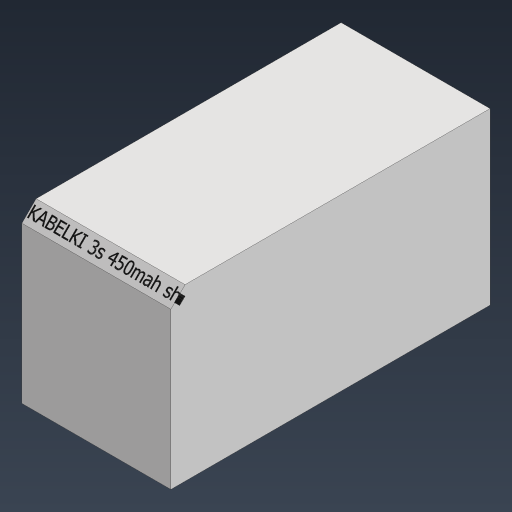
# Autodesk Inventor part: 2s450mah
Saved by Autodesk Inventor 2023 (Build 270158000, 158)
## iProperties
Created: 2026-03-09
Part Number: 2s450mah
Material: Generic
Document SubType Name: Modeling
Designer: szymo
Density: 1 g/cm^3
Appearance: Default
Author: szymo
Autodesk Inventor part; units mm, degrees
ref_plane "YZ Plane" through (0, 0, 0) normal (1, 0, 0) x (0, 1, 0)
ref_plane "XZ Plane" through (0, 0, 0) normal (0, 1, 0) x (-1, 0, 0)
ref_plane "XY Plane" through (0, 0, 0) normal (0, 0, 1) x (1, 0, 0)
sketch "Sketch1" plane through (0, 0, 0) normal (0, 1, 0) x (-1, 0, 0)
  line L0 (0, 0) -> (-21, 0)
  line L1 (-21, 0) -> (-21, -45)
  line L2 (-21, -45) -> (0, -45)
  line L3 (0, -45) -> (0, 0)
  dimension "d0" = 21
  dimension "d1" = 45
  constraints: 8 end point, 2 parallel, 1 horizontal, 1 perpendicular
  measures "d0" distance of L2.end L1.end
  measures "d1" distance of L0.end L1.end
extrude "Extrusion1" add sketch "Sketch1" along normal blind 24
chamfer "Chamfer1" distance 2 angle 45 1 edges at (10.5, 24, 0)
sketch "Sketch2" plane through (0, 24, -2) normal (0, 0.7071068, 0.7071068) x (1, 0, 0)
  line L0 (0.0469, -0.5129) -> (26.4473, -0.5129) construction
  line L1 (26.4473, -0.5129) -> (26.4473, -3.2591) construction
  line L2 (26.4473, -3.2591) -> (0.0469, -3.2591) construction
  line L3 (0.0469, -3.2591) -> (0.0469, -0.5129) construction
  line L4 (1.2929, -2.0798) -> (1.0339, -2.0798)
  line L5 (1.0339, -2.0798) -> (0.4857, -1.382)
  line L6 (0.4857, -1.382) -> (0.3982, -1.4805)
  line L7 (0.3982, -1.4805) -> (0.3982, -2.0798)
  line L8 (0.3982, -2.0798) -> (0.1989, -2.0798)
  line L9 (0.1989, -2.0798) -> (0.1989, -0.5798)
  line L10 (0.1989, -0.5798) -> (0.3982, -0.5798)
  line L11 (0.3982, -0.5798) -> (0.3982, -1.269)
  line L12 (0.3982, -1.269) -> (1.0133, -0.5798)
  line L13 (1.0133, -0.5798) -> (1.2564, -0.5798)
  line L14 (1.2564, -0.5798) -> (0.6352, -1.2495)
  line L15 (0.6352, -1.2495) -> (1.2929, -2.0798)
  line L16 (1.2503, -2.0798) -> (1.756, -0.5798)
  line L17 (1.756, -0.5798) -> (2.0015, -0.5798)
  line L18 (2.0015, -0.5798) -> (2.5072, -2.0798)
  line L19 (2.5072, -2.0798) -> (2.2969, -2.0798)
  line L20 (2.2969, -2.0798) -> (2.1608, -1.6604)
  line L21 (2.1608, -1.6604) -> (1.5882, -1.6604)
  line L22 (1.5882, -1.6604) -> (1.4521, -2.0798)
  line L23 (1.4521, -2.0798) -> (1.2503, -2.0798)
  line L24 (2.1061, -1.4902) -> (1.8739, -0.784)
  line L25 (1.8739, -0.784) -> (1.6429, -1.4902)
  line L26 (1.6429, -1.4902) -> (2.1061, -1.4902)
  spline S0 degree 2 poles (3.6668, -1.6191) (3.6668, -1.7309) (3.5818, -1.9023) (3.5113, -1.9582) knots 0 0 0 1 2 2 2
  spline S1 degree 2 poles (3.5113, -1.9582) (3.4262, -2.0238) (3.2329, -2.0798) (3.0797, -2.0798) knots 0 0 0 1 2 2 2
  line L27 (3.0797, -2.0798) -> (2.6494, -2.0798)
  line L28 (2.6494, -2.0798) -> (2.6494, -0.5798)
  line L29 (2.6494, -0.5798) -> (3.0469, -0.5798)
  spline S2 degree 2 poles (3.0469, -0.5798) (3.2074, -0.5798) (3.3678, -0.6004) (3.4407, -0.6405) knots 0 0 0 1 2 2 2
  spline S3 degree 2 poles (3.4407, -0.6405) (3.5222, -0.6831) (3.5963, -0.8229) (3.5963, -0.9177) knots 0 0 0 1 2 2 2
  spline S4 degree 2 poles (3.5963, -0.9177) (3.5963, -1.0234) (3.4845, -1.1912) (3.386, -1.2386) knots 0 0 0 1 2 2 2
  line L30 (3.386, -1.2386) -> (3.386, -1.2459)
  spline S5 degree 2 poles (3.386, -1.2459) (3.5198, -1.2824) (3.6668, -1.4756) (3.6668, -1.6191) knots 0 0 0 1 2 2 2
  spline S6 degree 2 poles (3.459, -1.6276) (3.459, -1.5425) (3.4104, -1.4331) (3.3374, -1.3942) knots 0 0 0 1 2 2 2
  spline S7 degree 2 poles (3.3374, -1.3942) (3.29, -1.3699) (3.1782, -1.3553) (3.0749, -1.3553) knots 0 0 0 1 2 2 2
  line L31 (3.0749, -1.3553) -> (2.8488, -1.3553)
  line L32 (2.8488, -1.3553) -> (2.8488, -1.9096)
  line L33 (2.8488, -1.9096) -> (3.0104, -1.9096)
  spline S8 degree 2 poles (3.0104, -1.9096) (3.1417, -1.9096) (3.2924, -1.8853) (3.3508, -1.8464) knots 0 0 0 1 2 2 2
  spline S9 degree 2 poles (3.3508, -1.8464) (3.4067, -1.8063) (3.459, -1.7066) (3.459, -1.6276) knots 0 0 0 1 2 2 2
  spline S10 degree 2 poles (3.3885, -0.9456) (3.3885, -0.8922) (3.352, -0.8119) (3.3119, -0.7888) knots 0 0 0 1 2 2 2
  spline S11 degree 2 poles (3.3119, -0.7888) (3.2633, -0.7621) (3.1454, -0.7499) (3.0396, -0.7499) knots 0 0 0 1 2 2 2
  line L34 (3.0396, -0.7499) -> (2.8488, -0.7499)
  line L35 (2.8488, -0.7499) -> (2.8488, -1.1888)
  line L36 (2.8488, -1.1888) -> (3.0749, -1.1888)
  spline S12 degree 2 poles (3.0749, -1.1888) (3.1685, -1.1888) (3.2572, -1.1693) (3.3046, -1.1389) knots 0 0 0 1 2 2 2
  spline S13 degree 2 poles (3.3046, -1.1389) (3.3508, -1.1097) (3.3885, -1.0161) (3.3885, -0.9456) knots 0 0 0 1 2 2 2
  line L37 (3.865, -2.0798) -> (3.865, -0.5798)
  line L38 (3.865, -0.5798) -> (4.8034, -0.5798)
  line L39 (4.8034, -0.5798) -> (4.8034, -0.7572)
  line L40 (4.8034, -0.7572) -> (4.0643, -0.7572)
  line L41 (4.0643, -0.7572) -> (4.0643, -1.1681)
  line L42 (4.0643, -1.1681) -> (4.7536, -1.1681)
  line L43 (4.7536, -1.1681) -> (4.7536, -1.3456)
  line L44 (4.7536, -1.3456) -> (4.0643, -1.3456)
  line L45 (4.0643, -1.3456) -> (4.0643, -1.9023)
  line L46 (4.0643, -1.9023) -> (4.8034, -1.9023)
  line L47 (4.8034, -1.9023) -> (4.8034, -2.0798)
  line L48 (4.8034, -2.0798) -> (3.865, -2.0798)
  line L49 (5.8913, -2.0798) -> (5.0222, -2.0798)
  line L50 (5.0222, -2.0798) -> (5.0222, -0.5798)
  line L51 (5.0222, -0.5798) -> (5.2215, -0.5798)
  line L52 (5.2215, -0.5798) -> (5.2215, -1.9023)
  line L53 (5.2215, -1.9023) -> (5.8913, -1.9023)
  line L54 (5.8913, -1.9023) -> (5.8913, -2.0798)
  line L55 (7.1421, -2.0798) -> (6.8832, -2.0798)
  line L56 (6.8832, -2.0798) -> (6.335, -1.382)
  line L57 (6.335, -1.382) -> (6.2475, -1.4805)
  line L58 (6.2475, -1.4805) -> (6.2475, -2.0798)
  line L59 (6.2475, -2.0798) -> (6.0481, -2.0798)
  line L60 (6.0481, -2.0798) -> (6.0481, -0.5798)
  line L61 (6.0481, -0.5798) -> (6.2475, -0.5798)
  line L62 (6.2475, -0.5798) -> (6.2475, -1.269)
  line L63 (6.2475, -1.269) -> (6.8625, -0.5798)
  line L64 (6.8625, -0.5798) -> (7.1057, -0.5798)
  line L65 (7.1057, -0.5798) -> (6.4845, -1.2495)
  line L66 (6.4845, -1.2495) -> (7.1421, -2.0798)
  line L67 (7.7839, -2.0798) -> (7.2029, -2.0798)
  line L68 (7.2029, -2.0798) -> (7.2029, -1.9266)
  line L69 (7.2029, -1.9266) -> (7.3937, -1.9266)
  line L70 (7.3937, -1.9266) -> (7.3937, -0.7329)
  line L71 (7.3937, -0.7329) -> (7.2029, -0.7329)
  line L72 (7.2029, -0.7329) -> (7.2029, -0.5798)
  line L73 (7.2029, -0.5798) -> (7.7839, -0.5798)
  line L74 (7.7839, -0.5798) -> (7.7839, -0.7329)
  line L75 (7.7839, -0.7329) -> (7.5931, -0.7329)
  line L76 (7.5931, -0.7329) -> (7.5931, -1.9266)
  line L77 (7.5931, -1.9266) -> (7.7839, -1.9266)
  line L78 (7.7839, -1.9266) -> (7.7839, -2.0798)
  spline S14 degree 2 poles (9.0372, -0.722) (8.9825, -0.722) (8.8743, -0.7487) (8.822, -0.7694) knots 0 0 0 1 2 2 2
  spline S15 degree 2 poles (8.822, -0.7694) (8.7734, -0.7901) (8.7017, -0.8338) (8.6737, -0.8533) knots 0 0 0 1 2 2 2
  line L79 (8.6737, -0.8533) -> (8.6616, -0.8533)
  line L80 (8.6616, -0.8533) -> (8.6616, -0.6405)
  spline S16 degree 2 poles (8.6616, -0.6405) (8.7272, -0.6053) (8.9521, -0.5482) (9.053, -0.5482) knots 0 0 0 1 2 2 2
  spline S17 degree 2 poles (9.053, -0.5482) (9.1551, -0.5482) (9.307, -0.5895) (9.369, -0.6332) knots 0 0 0 1 2 2 2
  spline S18 degree 2 poles (9.369, -0.6332) (9.4347, -0.6807) (9.5027, -0.818) (9.5027, -0.9104) knots 0 0 0 1 2 2 2
  spline S19 degree 2 poles (9.5027, -0.9104) (9.5027, -1.0344) (9.3399, -1.2216) (9.2256, -1.2459) knots 0 0 0 1 2 2 2
  line L81 (9.2256, -1.2459) -> (9.2256, -1.2605)
  spline S20 degree 2 poles (9.2256, -1.2605) (9.273, -1.2702) (9.3812, -1.314) (9.4274, -1.3577) knots 0 0 0 1 2 2 2
  spline S21 degree 2 poles (9.4274, -1.3577) (9.4736, -1.4003) (9.5319, -1.5364) (9.5319, -1.6349) knots 0 0 0 1 2 2 2
  spline S22 degree 2 poles (9.5319, -1.6349) (9.5319, -1.7358) (9.4626, -1.9072) (9.3994, -1.9728) knots 0 0 0 1 2 2 2
  spline S23 degree 2 poles (9.3994, -1.9728) (9.3338, -2.0409) (9.1478, -2.1114) (9.0299, -2.1114) knots 0 0 0 1 2 2 2
  spline S24 degree 2 poles (9.0299, -2.1114) (8.9168, -2.1114) (8.6956, -2.0567) (8.6202, -2.019) knots 0 0 0 1 2 2 2
  line L82 (8.6202, -2.019) -> (8.6202, -1.8063)
  line L83 (8.6202, -1.8063) -> (8.6348, -1.8063)
  spline S25 degree 2 poles (8.6348, -1.8063) (8.698, -1.8525) (8.912, -1.9375) (9.0177, -1.9375) knots 0 0 0 1 2 2 2
  spline S26 degree 2 poles (9.0177, -1.9375) (9.0797, -1.9375) (9.2037, -1.8986) (9.245, -1.8537) knots 0 0 0 1 2 2 2
  spline S27 degree 2 poles (9.245, -1.8537) (9.2852, -1.8087) (9.3277, -1.7017) (9.3277, -1.6203) knots 0 0 0 1 2 2 2
  spline S28 degree 2 poles (9.3277, -1.6203) (9.3277, -1.5388) (9.2803, -1.4331) (9.2377, -1.4027) knots 0 0 0 1 2 2 2
  spline S29 degree 2 poles (9.2377, -1.4027) (9.1952, -1.3723) (9.0797, -1.3492) (9.0117, -1.3492) knots 0 0 0 1 2 2 2
  line L84 (9.0117, -1.3492) -> (8.9266, -1.3492)
  line L85 (8.9266, -1.3492) -> (8.9266, -1.1827)
  line L86 (8.9266, -1.1827) -> (8.9934, -1.1827)
  spline S30 degree 2 poles (8.9934, -1.1827) (9.1283, -1.1827) (9.2985, -1.0538) (9.2985, -0.9311) knots 0 0 0 1 2 2 2
  spline S31 degree 2 poles (9.2985, -0.9311) (9.2985, -0.8739) (9.2548, -0.7925) (9.2195, -0.7682) knots 0 0 0 1 2 2 2
  spline S32 degree 2 poles (9.2195, -0.7682) (9.1818, -0.7426) (9.0895, -0.722) (9.0372, -0.722) knots 0 0 0 1 2 2 2
  spline S33 degree 2 poles (10.0899, -2.1065) (9.9768, -2.1065) (9.7811, -2.0457) (9.7167, -2.0117) knots 0 0 0 1 2 2 2
  line L87 (9.7167, -2.0117) -> (9.7167, -1.799)
  line L88 (9.7167, -1.799) -> (9.7264, -1.799)
  spline S34 degree 2 poles (9.7264, -1.799) (9.7507, -1.8184) (9.8164, -1.8646) (9.8711, -1.8901) knots 0 0 0 1 2 2 2
  spline S35 degree 2 poles (9.8711, -1.8901) (9.9185, -1.9132) (10.0352, -1.9473) (10.0971, -1.9473) knots 0 0 0 1 2 2 2
  spline S36 degree 2 poles (10.0971, -1.9473) (10.1421, -1.9473) (10.2454, -1.9266) (10.2698, -1.9096) knots 0 0 0 1 2 2 2
  spline S37 degree 2 poles (10.2698, -1.9096) (10.305, -1.8865) (10.3366, -1.8342) (10.3366, -1.7807) knots 0 0 0 1 2 2 2
  spline S38 degree 2 poles (10.3366, -1.7807) (10.3366, -1.7139) (10.2637, -1.6446) (10.1701, -1.6215) knots 0 0 0 1 2 2 2
  spline S39 degree 2 poles (10.1701, -1.6215) (10.1336, -1.613) (10.0169, -1.5887) (9.9671, -1.5753) knots 0 0 0 1 2 2 2
  spline S40 degree 2 poles (9.9671, -1.5753) (9.8382, -1.5376) (9.7215, -1.382) (9.7215, -1.2714) knots 0 0 0 1 2 2 2
  spline S41 degree 2 poles (9.7215, -1.2714) (9.7215, -1.1183) (9.9513, -0.9274) (10.1409, -0.9274) knots 0 0 0 1 2 2 2
  spline S42 degree 2 poles (10.1409, -0.9274) (10.2345, -0.9274) (10.4241, -0.9736) (10.4886, -1.0089) knots 0 0 0 1 2 2 2
  line L89 (10.4886, -1.0089) -> (10.4886, -1.2119)
  line L90 (10.4886, -1.2119) -> (10.4788, -1.2119)
  spline S43 degree 2 poles (10.4788, -1.2119) (10.4059, -1.1535) (10.2284, -1.0867) (10.1373, -1.0867) knots 0 0 0 1 2 2 2
  spline S44 degree 2 poles (10.1373, -1.0867) (10.0437, -1.0867) (9.9148, -1.1657) (9.9148, -1.2447) knots 0 0 0 1 2 2 2
  spline S45 degree 2 poles (9.9148, -1.2447) (9.9148, -1.3164) (9.9914, -1.3857) (10.0765, -1.4076) knots 0 0 0 1 2 2 2
  spline S46 degree 2 poles (10.0765, -1.4076) (10.1178, -1.4185) (10.2224, -1.4404) (10.2795, -1.4538) knots 0 0 0 1 2 2 2
  spline S47 degree 2 poles (10.2795, -1.4538) (10.4035, -1.4854) (10.5299, -1.63) (10.5299, -1.7552) knots 0 0 0 1 2 2 2
  spline S48 degree 2 poles (10.5299, -1.7552) (10.5299, -1.8281) (10.4728, -1.957) (10.4168, -2.0044) knots 0 0 0 1 2 2 2
  spline S49 degree 2 poles (10.4168, -2.0044) (10.3573, -2.0542) (10.2053, -2.1065) (10.0899, -2.1065) knots 0 0 0 1 2 2 2
  line L91 (12.2876, -1.5644) -> (12.1089, -1.5644)
  line L92 (12.1089, -1.5644) -> (12.1089, -2.0798)
  line L93 (12.1089, -2.0798) -> (11.9156, -2.0798)
  line L94 (11.9156, -2.0798) -> (11.9156, -1.5644)
  line L95 (11.9156, -1.5644) -> (11.2531, -1.5644)
  line L96 (11.2531, -1.5644) -> (11.2531, -1.3529)
  line L97 (11.2531, -1.3529) -> (11.9241, -0.5798)
  line L98 (11.9241, -0.5798) -> (12.1089, -0.5798)
  line L99 (12.1089, -0.5798) -> (12.1089, -1.4027)
  line L100 (12.1089, -1.4027) -> (12.2876, -1.4027)
  line L101 (12.2876, -1.4027) -> (12.2876, -1.5644)
  line L102 (11.9156, -1.4027) -> (11.9156, -0.8168)
  line L103 (11.9156, -0.8168) -> (11.4112, -1.4027)
  line L104 (11.4112, -1.4027) -> (11.9156, -1.4027)
  spline S50 degree 2 poles (13.3573, -1.6033) (13.3573, -1.7114) (13.288, -1.8962) (13.2248, -1.9643) knots 0 0 0 1 2 2 2
  spline S51 degree 2 poles (13.2248, -1.9643) (13.1616, -2.0324) (12.9732, -2.1114) (12.8565, -2.1114) knots 0 0 0 1 2 2 2
  spline S52 degree 2 poles (12.8565, -2.1114) (12.7495, -2.1114) (12.5404, -2.064) (12.4638, -2.0263) knots 0 0 0 1 2 2 2
  line L105 (12.4638, -2.0263) -> (12.4638, -1.8136)
  line L106 (12.4638, -1.8136) -> (12.4784, -1.8136)
  spline S53 degree 2 poles (12.4784, -1.8136) (12.5015, -1.8306) (12.5878, -1.8743) (12.6401, -1.8938) knots 0 0 0 1 2 2 2
  spline S54 degree 2 poles (12.6401, -1.8938) (12.6997, -1.9144) (12.7981, -1.9375) (12.8601, -1.9375) knots 0 0 0 1 2 2 2
  spline S55 degree 2 poles (12.8601, -1.9375) (12.9209, -1.9375) (13.0352, -1.8938) (13.0765, -1.8464) knots 0 0 0 1 2 2 2
  spline S56 degree 2 poles (13.0765, -1.8464) (13.1142, -1.8014) (13.1531, -1.6823) (13.1531, -1.602) knots 0 0 0 1 2 2 2
  spline S57 degree 2 poles (13.1531, -1.602) (13.1531, -1.5218) (13.1093, -1.4197) (13.068, -1.3857) knots 0 0 0 1 2 2 2
  spline S58 degree 2 poles (13.068, -1.3857) (13.0254, -1.348) (12.899, -1.3164) (12.8224, -1.3164) knots 0 0 0 1 2 2 2
  spline S59 degree 2 poles (12.8224, -1.3164) (12.7398, -1.3164) (12.5757, -1.3419) (12.5258, -1.3529) knots 0 0 0 1 2 2 2
  line L107 (12.5258, -1.3529) -> (12.5258, -0.5798)
  line L108 (12.5258, -0.5798) -> (13.3488, -0.5798)
  line L109 (13.3488, -0.5798) -> (13.3488, -0.756)
  line L110 (13.3488, -0.756) -> (12.7191, -0.756)
  line L111 (12.7191, -0.756) -> (12.7191, -1.1559)
  spline S60 degree 2 poles (12.7191, -1.1559) (12.7556, -1.1511) (12.8261, -1.1474) (12.8553, -1.1474) knots 0 0 0 1 2 2 2
  spline S61 degree 2 poles (12.8553, -1.1474) (12.9707, -1.1474) (13.13, -1.1851) (13.2029, -1.241) knots 0 0 0 1 2 2 2
  spline S62 degree 2 poles (13.2029, -1.241) (13.2771, -1.2969) (13.3573, -1.4671) (13.3573, -1.6033) knots 0 0 0 1 2 2 2
  spline S63 degree 2 poles (14.5072, -1.3298) (14.5072, -1.7333) (14.2726, -2.1114) (14.0283, -2.1114) knots 0 0 0 1 2 2 2
  spline S64 degree 2 poles (14.0283, -2.1114) (13.7803, -2.1114) (13.5481, -1.726) (13.5481, -1.331) knots 0 0 0 1 2 2 2
  spline S65 degree 2 poles (13.5481, -1.331) (13.5481, -0.925) (13.7827, -0.5494) (14.0283, -0.5494) knots 0 0 0 1 2 2 2
  spline S66 degree 2 poles (14.0283, -0.5494) (14.275, -0.5494) (14.5072, -0.9384) (14.5072, -1.3298) knots 0 0 0 1 2 2 2
  spline S67 degree 2 poles (14.2495, -1.7868) (14.2787, -1.7127) (14.303, -1.4841) (14.303, -1.3298) knots 0 0 0 1 2 2 2
  spline S68 degree 2 poles (14.303, -1.3298) (14.303, -1.1754) (14.2787, -0.9481) (14.2483, -0.8715) knots 0 0 0 1 2 2 2
  spline S69 degree 2 poles (14.2483, -0.8715) (14.2179, -0.7949) (14.1121, -0.7159) (14.0283, -0.7159) knots 0 0 0 1 2 2 2
  spline S70 degree 2 poles (14.0283, -0.7159) (13.9444, -0.7159) (13.8362, -0.7949) (13.8046, -0.8739) knots 0 0 0 1 2 2 2
  spline S71 degree 2 poles (13.8046, -0.8739) (13.7742, -0.9505) (13.7523, -1.1839) (13.7523, -1.331) knots 0 0 0 1 2 2 2
  spline S72 degree 2 poles (13.7523, -1.331) (13.7523, -1.489) (13.7718, -1.7005) (13.8034, -1.7832) knots 0 0 0 1 2 2 2
  spline S73 degree 2 poles (13.8034, -1.7832) (13.8326, -1.861) (13.9407, -1.9448) (14.0283, -1.9448) knots 0 0 0 1 2 2 2
  spline S74 degree 2 poles (14.0283, -1.9448) (14.1109, -1.9448) (14.2191, -1.8658) (14.2495, -1.7868) knots 0 0 0 1 2 2 2
  line L112 (16.0036, -2.0798) -> (16.0036, -1.4282)
  spline S75 degree 2 poles (16.0036, -1.4282) (16.0036, -1.3504) (15.9914, -1.2179) (15.9719, -1.1815) knots 0 0 0 1 2 2 2
  spline S76 degree 2 poles (15.9719, -1.1815) (15.9525, -1.1414) (15.8783, -1.1025) (15.8139, -1.1025) knots 0 0 0 1 2 2 2
  spline S77 degree 2 poles (15.8139, -1.1025) (15.7556, -1.1025) (15.6219, -1.1742) (15.5514, -1.2422) knots 0 0 0 1 2 2 2
  spline S78 degree 2 poles (15.5514, -1.2422) (15.5526, -1.2593) (15.555, -1.3067) (15.555, -1.3383) knots 0 0 0 1 2 2 2
  line L113 (15.555, -1.3383) -> (15.555, -2.0798)
  line L114 (15.555, -2.0798) -> (15.3654, -2.0798)
  line L115 (15.3654, -2.0798) -> (15.3654, -1.4282)
  spline S79 degree 2 poles (15.3654, -1.4282) (15.3654, -1.3504) (15.3532, -1.2179) (15.3338, -1.1815) knots 0 0 0 1 2 2 2
  spline S80 degree 2 poles (15.3338, -1.1815) (15.3143, -1.1414) (15.2402, -1.1025) (15.1758, -1.1025) knots 0 0 0 1 2 2 2
  spline S81 degree 2 poles (15.1758, -1.1025) (15.115, -1.1025) (14.9801, -1.179) (14.9168, -1.2386) knots 0 0 0 1 2 2 2
  line L116 (14.9168, -1.2386) -> (14.9168, -2.0798)
  line L117 (14.9168, -2.0798) -> (14.7272, -2.0798)
  line L118 (14.7272, -2.0798) -> (14.7272, -0.9542)
  line L119 (14.7272, -0.9542) -> (14.9168, -0.9542)
  line L120 (14.9168, -0.9542) -> (14.9168, -1.0781)
  spline S82 degree 2 poles (14.9168, -1.0781) (14.991, -1.004) (15.1369, -0.9226) (15.2244, -0.9226) knots 0 0 0 1 2 2 2
  spline S83 degree 2 poles (15.2244, -0.9226) (15.3241, -0.9226) (15.4784, -1.0137) (15.5185, -1.117) knots 0 0 0 1 2 2 2
  spline S84 degree 2 poles (15.5185, -1.117) (15.6048, -1.021) (15.7677, -0.9226) (15.8625, -0.9226) knots 0 0 0 1 2 2 2
  spline S85 degree 2 poles (15.8625, -0.9226) (15.9355, -0.9226) (16.0546, -0.9675) (16.0984, -1.0186) knots 0 0 0 1 2 2 2
  spline S86 degree 2 poles (16.0984, -1.0186) (16.1433, -1.0696) (16.1932, -1.2228) (16.1932, -1.3383) knots 0 0 0 1 2 2 2
  line L121 (16.1932, -1.3383) -> (16.1932, -2.0798)
  line L122 (16.1932, -2.0798) -> (16.0036, -2.0798)
  spline S87 degree 2 poles (17.0866, -1.9606) (17.0635, -1.9777) (16.9857, -2.0384) (16.9493, -2.0567) knots 0 0 0 1 2 2 2
  spline S88 degree 2 poles (16.9493, -2.0567) (16.8994, -2.0834) (16.8058, -2.1114) (16.7207, -2.1114) knots 0 0 0 1 2 2 2
  spline S89 degree 2 poles (16.7207, -2.1114) (16.6514, -2.1114) (16.5262, -2.0591) (16.4788, -2.0117) knots 0 0 0 1 2 2 2
  spline S90 degree 2 poles (16.4788, -2.0117) (16.4339, -1.9655) (16.3792, -1.8294) (16.3792, -1.754) knots 0 0 0 1 2 2 2
  spline S91 degree 2 poles (16.3792, -1.754) (16.3792, -1.6373) (16.4776, -1.472) (16.5846, -1.4246) knots 0 0 0 1 2 2 2
  spline S92 degree 2 poles (16.5846, -1.4246) (16.6794, -1.3808) (16.9371, -1.348) (17.0866, -1.3395) knots 0 0 0 1 2 2 2
  line L123 (17.0866, -1.3395) -> (17.0866, -1.303)
  spline S93 degree 2 poles (17.0866, -1.303) (17.0866, -1.2374) (17.0465, -1.1559) (17.01, -1.1328) knots 0 0 0 1 2 2 2
  spline S94 degree 2 poles (17.01, -1.1328) (16.9736, -1.1097) (16.869, -1.0952) (16.8131, -1.0952) knots 0 0 0 1 2 2 2
  spline S95 degree 2 poles (16.8131, -1.0952) (16.7475, -1.0952) (16.57, -1.1341) (16.4813, -1.1717) knots 0 0 0 1 2 2 2
  line L124 (16.4813, -1.1717) -> (16.4703, -1.1717)
  line L125 (16.4703, -1.1717) -> (16.4703, -0.9785)
  spline S96 degree 2 poles (16.4703, -0.9785) (16.5226, -0.9639) (16.7183, -0.9274) (16.8143, -0.9274) knots 0 0 0 1 2 2 2
  spline S97 degree 2 poles (16.8143, -0.9274) (16.931, -0.9274) (17.0903, -0.9639) (17.1535, -1.0113) knots 0 0 0 1 2 2 2
  spline S98 degree 2 poles (17.1535, -1.0113) (17.2155, -1.0575) (17.2762, -1.2046) (17.2762, -1.3103) knots 0 0 0 1 2 2 2
  line L126 (17.2762, -1.3103) -> (17.2762, -2.0798)
  line L127 (17.2762, -2.0798) -> (17.0866, -2.0798)
  line L128 (17.0866, -2.0798) -> (17.0866, -1.9606)
  line L129 (17.0866, -1.8026) -> (17.0866, -1.4902)
  spline S99 degree 2 poles (17.0866, -1.4902) (17.0185, -1.4963) (16.8131, -1.517) (16.7487, -1.5364) knots 0 0 0 1 2 2 2
  spline S100 degree 2 poles (16.7487, -1.5364) (16.6733, -1.5595) (16.5749, -1.6555) (16.5749, -1.7406) knots 0 0 0 1 2 2 2
  spline S101 degree 2 poles (16.5749, -1.7406) (16.5749, -1.8379) (16.6843, -1.9363) (16.7888, -1.9363) knots 0 0 0 1 2 2 2
  spline S102 degree 2 poles (16.7888, -1.9363) (16.8775, -1.9363) (17.0234, -1.8597) (17.0866, -1.8026) knots 0 0 0 1 2 2 2
  line L130 (18.4262, -2.0798) -> (18.2365, -2.0798)
  line L131 (18.2365, -2.0798) -> (18.2365, -1.4379)
  spline S103 degree 2 poles (18.2365, -1.4379) (18.2365, -1.3602) (18.2219, -1.2264) (18.2001, -1.1863) knots 0 0 0 1 2 2 2
  spline S104 degree 2 poles (18.2001, -1.1863) (18.177, -1.1438) (18.0943, -1.1025) (18.0238, -1.1025) knots 0 0 0 1 2 2 2
  spline S105 degree 2 poles (18.0238, -1.1025) (17.9533, -1.1025) (17.8038, -1.1778) (17.7321, -1.2386) knots 0 0 0 1 2 2 2
  line L132 (17.7321, -1.2386) -> (17.7321, -2.0798)
  line L133 (17.7321, -2.0798) -> (17.5425, -2.0798)
  line L134 (17.5425, -2.0798) -> (17.5425, -0.5129)
  line L135 (17.5425, -0.5129) -> (17.7321, -0.5129)
  line L136 (17.7321, -0.5129) -> (17.7321, -1.0794)
  spline S106 degree 2 poles (17.7321, -1.0794) (17.8172, -1.0028) (17.9813, -0.9226) (18.0736, -0.9226) knots 0 0 0 1 2 2 2
  spline S107 degree 2 poles (18.0736, -0.9226) (18.239, -0.9226) (18.4262, -1.1414) (18.4262, -1.3492) knots 0 0 0 1 2 2 2
  line L137 (18.4262, -1.3492) -> (18.4262, -2.0798)
  spline S108 degree 2 poles (19.6405, -2.1065) (19.5275, -2.1065) (19.3318, -2.0457) (19.2673, -2.0117) knots 0 0 0 1 2 2 2
  line L138 (19.2673, -2.0117) -> (19.2673, -1.799)
  line L139 (19.2673, -1.799) -> (19.2771, -1.799)
  spline S109 degree 2 poles (19.2771, -1.799) (19.3014, -1.8184) (19.367, -1.8646) (19.4217, -1.8901) knots 0 0 0 1 2 2 2
  spline S110 degree 2 poles (19.4217, -1.8901) (19.4691, -1.9132) (19.5858, -1.9473) (19.6478, -1.9473) knots 0 0 0 1 2 2 2
  spline S111 degree 2 poles (19.6478, -1.9473) (19.6928, -1.9473) (19.7961, -1.9266) (19.8204, -1.9096) knots 0 0 0 1 2 2 2
  spline S112 degree 2 poles (19.8204, -1.9096) (19.8557, -1.8865) (19.8873, -1.8342) (19.8873, -1.7807) knots 0 0 0 1 2 2 2
  spline S113 degree 2 poles (19.8873, -1.7807) (19.8873, -1.7139) (19.8143, -1.6446) (19.7207, -1.6215) knots 0 0 0 1 2 2 2
  spline S114 degree 2 poles (19.7207, -1.6215) (19.6843, -1.613) (19.5676, -1.5887) (19.5177, -1.5753) knots 0 0 0 1 2 2 2
  spline S115 degree 2 poles (19.5177, -1.5753) (19.3889, -1.5376) (19.2722, -1.382) (19.2722, -1.2714) knots 0 0 0 1 2 2 2
  spline S116 degree 2 poles (19.2722, -1.2714) (19.2722, -1.1183) (19.5019, -0.9274) (19.6916, -0.9274) knots 0 0 0 1 2 2 2
  spline S117 degree 2 poles (19.6916, -0.9274) (19.7852, -0.9274) (19.9748, -0.9736) (20.0392, -1.0089) knots 0 0 0 1 2 2 2
  line L140 (20.0392, -1.0089) -> (20.0392, -1.2119)
  line L141 (20.0392, -1.2119) -> (20.0295, -1.2119)
  spline S118 degree 2 poles (20.0295, -1.2119) (19.9566, -1.1535) (19.7791, -1.0867) (19.6879, -1.0867) knots 0 0 0 1 2 2 2
  spline S119 degree 2 poles (19.6879, -1.0867) (19.5943, -1.0867) (19.4655, -1.1657) (19.4655, -1.2447) knots 0 0 0 1 2 2 2
  spline S120 degree 2 poles (19.4655, -1.2447) (19.4655, -1.3164) (19.542, -1.3857) (19.6271, -1.4076) knots 0 0 0 1 2 2 2
  spline S121 degree 2 poles (19.6271, -1.4076) (19.6685, -1.4185) (19.773, -1.4404) (19.8301, -1.4538) knots 0 0 0 1 2 2 2
  spline S122 degree 2 poles (19.8301, -1.4538) (19.9541, -1.4854) (20.0805, -1.63) (20.0805, -1.7552) knots 0 0 0 1 2 2 2
  spline S123 degree 2 poles (20.0805, -1.7552) (20.0805, -1.8281) (20.0234, -1.957) (19.9675, -2.0044) knots 0 0 0 1 2 2 2
  spline S124 degree 2 poles (19.9675, -2.0044) (19.9079, -2.0542) (19.756, -2.1065) (19.6405, -2.1065) knots 0 0 0 1 2 2 2
  line L142 (21.1405, -2.0798) -> (20.9509, -2.0798)
  line L143 (20.9509, -2.0798) -> (20.9509, -1.4379)
  spline S125 degree 2 poles (20.9509, -1.4379) (20.9509, -1.3602) (20.9363, -1.2264) (20.9144, -1.1863) knots 0 0 0 1 2 2 2
  spline S126 degree 2 poles (20.9144, -1.1863) (20.8913, -1.1438) (20.8087, -1.1025) (20.7382, -1.1025) knots 0 0 0 1 2 2 2
  spline S127 degree 2 poles (20.7382, -1.1025) (20.6677, -1.1025) (20.5181, -1.1778) (20.4464, -1.2386) knots 0 0 0 1 2 2 2
  line L144 (20.4464, -1.2386) -> (20.4464, -2.0798)
  line L145 (20.4464, -2.0798) -> (20.2568, -2.0798)
  line L146 (20.2568, -2.0798) -> (20.2568, -0.5129)
  line L147 (20.2568, -0.5129) -> (20.4464, -0.5129)
  line L148 (20.4464, -0.5129) -> (20.4464, -1.0794)
  spline S128 degree 2 poles (20.4464, -1.0794) (20.5315, -1.0028) (20.6956, -0.9226) (20.788, -0.9226) knots 0 0 0 1 2 2 2
  spline S129 degree 2 poles (20.788, -0.9226) (20.9533, -0.9226) (21.1405, -1.1414) (21.1405, -1.3492) knots 0 0 0 1 2 2 2
  line L149 (21.1405, -1.3492) -> (21.1405, -2.0798)
  spline S130 degree 2 poles (22.3318, -1.517) (22.3318, -1.8014) (22.0583, -2.1114) (21.8297, -2.1114) knots 0 0 0 1 2 2 2
  spline S131 degree 2 poles (21.8297, -2.1114) (21.5951, -2.1114) (21.3265, -1.7917) (21.3265, -1.517) knots 0 0 0 1 2 2 2
  spline S132 degree 2 poles (21.3265, -1.517) (21.3265, -1.235) (21.6036, -0.9226) (21.8297, -0.9226) knots 0 0 0 1 2 2 2
  spline S133 degree 2 poles (21.8297, -0.9226) (22.0583, -0.9226) (22.3318, -1.2337) (22.3318, -1.517) knots 0 0 0 1 2 2 2
  spline S134 degree 2 poles (22.136, -1.517) (22.136, -1.2982) (21.9768, -1.0854) (21.8297, -1.0854) knots 0 0 0 1 2 2 2
  spline S135 degree 2 poles (21.8297, -1.0854) (21.6826, -1.0854) (21.5222, -1.2982) (21.5222, -1.517) knots 0 0 0 1 2 2 2
  spline S136 degree 2 poles (21.5222, -1.517) (21.5222, -1.7297) (21.6826, -1.9485) (21.8297, -1.9485) knots 0 0 0 1 2 2 2
  spline S137 degree 2 poles (21.8297, -1.9485) (21.9756, -1.9485) (22.136, -1.7333) (22.136, -1.517) knots 0 0 0 1 2 2 2
  line L150 (23.1231, -1.1572) -> (23.1134, -1.1572)
  spline S138 degree 2 poles (23.1134, -1.1572) (23.0915, -1.1511) (23.0441, -1.1486) (23.0113, -1.1486) knots 0 0 0 1 2 2 2
  spline S139 degree 2 poles (23.0113, -1.1486) (22.9347, -1.1486) (22.7839, -1.2155) (22.7159, -1.2811) knots 0 0 0 1 2 2 2
  line L151 (22.7159, -1.2811) -> (22.7159, -2.0798)
  line L152 (22.7159, -2.0798) -> (22.5262, -2.0798)
  line L153 (22.5262, -2.0798) -> (22.5262, -0.9542)
  line L154 (22.5262, -0.9542) -> (22.7159, -0.9542)
  line L155 (22.7159, -0.9542) -> (22.7159, -1.1219)
  spline S140 degree 2 poles (22.7159, -1.1219) (22.8192, -1.0295) (22.9736, -0.9542) (23.0465, -0.9542) knots 0 0 0 1 2 2 2
  spline S141 degree 2 poles (23.0465, -0.9542) (23.0757, -0.9542) (23.1048, -0.9566) (23.1231, -0.9602) knots 0 0 0 1 2 2 2
  line L156 (23.1231, -0.9602) -> (23.1231, -1.1572)
  spline S142 degree 2 poles (23.6105, -2.1016) (23.4561, -2.1016) (23.2823, -1.9254) (23.2823, -1.7345) knots 0 0 0 1 2 2 2
  line L157 (23.2823, -1.7345) -> (23.2823, -1.111)
  line L158 (23.2823, -1.111) -> (23.1547, -1.111)
  line L159 (23.1547, -1.111) -> (23.1547, -0.9542)
  line L160 (23.1547, -0.9542) -> (23.2823, -0.9542)
  line L161 (23.2823, -0.9542) -> (23.2823, -0.6308)
  line L162 (23.2823, -0.6308) -> (23.4719, -0.6308)
  line L163 (23.4719, -0.6308) -> (23.4719, -0.9542)
  line L164 (23.4719, -0.9542) -> (23.8208, -0.9542)
  line L165 (23.8208, -0.9542) -> (23.8208, -1.111)
  line L166 (23.8208, -1.111) -> (23.4719, -1.111)
  line L167 (23.4719, -1.111) -> (23.4719, -1.647)
  spline S143 degree 2 poles (23.4719, -1.647) (23.4719, -1.7321) (23.478, -1.8257) (23.4987, -1.8658) knots 0 0 0 1 2 2 2
  spline S144 degree 2 poles (23.4987, -1.8658) (23.5157, -1.9011) (23.5923, -1.9363) (23.6579, -1.9363) knots 0 0 0 1 2 2 2
  spline S145 degree 2 poles (23.6579, -1.9363) (23.7041, -1.9363) (23.7904, -1.9084) (23.8099, -1.8999) knots 0 0 0 1 2 2 2
  line L168 (23.8099, -1.8999) -> (23.8208, -1.8999)
  line L169 (23.8208, -1.8999) -> (23.8208, -2.07)
  spline S146 degree 2 poles (23.8208, -2.07) (23.7673, -2.0846) (23.6579, -2.1016) (23.6105, -2.1016) knots 0 0 0 1 2 2 2
  point P0 (0, -18.3848)
  constraints: 2 other
extrude "Extrusion2" cut sketch "Sketch2" against normal blind 1
body "Solid1"
